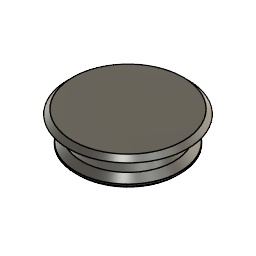
Stopfen_S-Max (Autodesk Fusion 360 design; units mm, degrees)
Autodesk Fusion 360 part; units mm, degrees
sketch "Skizze1" plane through (0, 0, 0) normal (0, 0, 1) x (1, 0, 0)
  circle A0 centre (0, 0) radius 30.8
  dimension "d1" = 61.6
  constraint coincident A0.centre origin
  measures "d1" diameter of A0
extrude "Extrusion1" add sketch "Skizze1" along normal blind 12
sketch "Skizze2" plane through (0, 0, 12) normal (0, 0, 1) x (-1, 0, 0)
  circle A0 centre (0, 0) radius 30.8
  circle A1 centre (0, 0) radius 40
  dimension "d4" = 80
  constraint coincident A0.centre A1.centre
  measures "d4" diameter of A1
extrude "Extrusion2" add sketch "Skizze2" along normal blind 3 contours A0 | A1
extrude "Extrusion4" add 1 faces at (6.9618, -9.4552, 0) along direction (0, 0, -1) blind 4
sketch "Skizze4" plane through (0, 0, -4) normal (0, 0, -1) x (1, 0, 0)
  circle A0 centre (0, 0) radius 30.8
  circle A1 centre (0, 0) radius 35
  dimension "d14" = 70
  constraint concentric A0 A1
  measures "d14" diameter of A1
extrude "Extrusion5" add sketch "Skizze4" along normal blind 3 contours A0 | A1
chamfer "Fase3" distance 2 angle 45 1 edges at (-32.6315, 12.6565, -7)
chamfer "Fase5" distance 3 angle 45 1 edges at (37.2931, 14.4646, 15)
sketch "Skizze5" plane through (0, 0, 15) normal (0, 0, 1) x (-1, 0, 0)
  circle A0 centre (0, 0) radius 37
  circle A1 centre (0, 0) radius 27
  dimension "d20" = 54
  constraint concentric A0 A1
  measures "d20" diameter of A1
chamfer "Fase7" distance 4 angle 45 1 edges at (-28.7157, 11.1378, -4)
